Autodesk Fusion 360 part; units mm, degrees
(part 4 of 24)
  arc A1417 (34.9504, 19.1008) -> (35.0012, 19.1008) centre (34.9758, 19.1008) ccw
  arc A1418 (30.7467, 19.1982) -> (30.7975, 19.1982) centre (30.7721, 19.1982) ccw
  arc A1419 (40.8996, 22.1629) -> (40.8996, 22.2137) centre (40.8996, 22.1883) ccw
  arc A1420 (27.3478, 19.5144) -> (27.3638, 19.4662) centre (27.3558, 19.4903) ccw
  arc A1421 (32.4358, 19.1262) -> (32.4358, 19.0754) centre (32.4358, 19.1008) ccw
  arc A1422 (32.4104, 19.4254) -> (32.4612, 19.4254) centre (32.4358, 19.4254) ccw
  arc A1423 (32.8253, 20.2819) -> (33.0849, 20.5415) centre (32.8253, 20.5415) ccw
  line L436 (33.6042, 19.1008) -> (32.4358, 19.1008)
  arc A1424 (29.8878, 19.5144) -> (29.9038, 19.4662) centre (29.8958, 19.4903) ccw
  arc A1425 (32.8253, 20.3073) -> (32.8253, 20.2565) centre (32.8253, 20.2819) ccw
  arc A1426 (33.1103, 20.5415) -> (33.0595, 20.5415) centre (33.0849, 20.5415) ccw
  arc A1427 (32.8253, 20.2565) -> (32.8253, 20.3073) centre (32.8253, 20.2819) ccw
  line L437 (40.0558, 21.5392) -> (40.0558, 21.8637)
  arc A1428 (31.0642, 20.6333) -> (30.4151, 20.6333) centre (30.7396, 20.6333) ccw
  line L438 (31.0642, 20.3087) -> (31.0642, 20.6333)
  line L439 (33.6042, 19.4254) -> (33.6042, 19.1008)
  arc A1429 (27.3558, 20.6657) -> (27.6154, 20.3087) centre (27.731, 20.6657) ccw
  line L440 (41.2242, 21.8637) -> (41.2242, 21.5392)
  line L441 (29.8958, 19.4903) -> (31.0642, 19.8797)
  line L442 (30.4151, 20.6982) -> (30.4151, 20.4385)
  arc A1430 (31.0388, 20.6333) -> (31.0896, 20.6333) centre (31.0642, 20.6333) ccw
  arc A1431 (30.4405, 20.6982) -> (30.3897, 20.6982) centre (30.4151, 20.6982) ccw
  arc A1432 (33.6042, 19.4254) -> (33.2796, 19.7499) centre (33.2796, 19.4253) ccw
  arc A1433 (33.0595, 20.5415) -> (33.1103, 20.5415) centre (33.0849, 20.5415) ccw
  arc A1434 (32.7604, 19.7499) -> (32.4358, 19.4254) centre (32.7604, 19.4253) ccw
  arc A1435 (40.0304, 21.5392) -> (40.0812, 21.5392) centre (40.0558, 21.5392) ccw
  arc A1436 (30.4151, 20.6982) -> (29.8958, 20.6982) centre (30.1554, 20.6982) ccw
  arc A1437 (32.7604, 20.3073) -> (32.7604, 20.2565) centre (32.7604, 20.2819) ccw
  line L443 (32.7604, 19.7499) -> (33.2796, 19.7499)
  arc A1438 (33.5788, 19.1008) -> (33.6296, 19.1008) centre (33.6042, 19.1008) ccw
  line L444 (34.9758, 19.1008) -> (34.9758, 19.4254)
  arc A1439 (31.0722, 19.8556) -> (31.0562, 19.9038) centre (31.0642, 19.8797) ccw
  arc A1440 (30.3897, 20.6982) -> (30.4405, 20.6982) centre (30.4151, 20.6982) ccw
  arc A1441 (28.5496, 20.9578) -> (28.4988, 20.9578) centre (28.5242, 20.9578) ccw
  arc A1442 (33.2796, 19.7753) -> (33.2796, 19.7245) centre (33.2796, 19.7499) ccw
  arc A1443 (29.8704, 20.6982) -> (29.9212, 20.6982) centre (29.8958, 20.6982) ccw
  arc A1444 (32.4104, 19.1008) -> (32.4612, 19.1008) centre (32.4358, 19.1008) ccw
  arc A1445 (32.7604, 19.7245) -> (32.7604, 19.7753) centre (32.7604, 19.7499) ccw
  arc A1446 (33.0849, 20.9056) -> (33.0849, 20.9564) centre (33.0849, 20.931) ccw
  arc A1447 (29.8704, 20.3087) -> (29.9212, 20.3087) centre (29.8958, 20.3087) ccw
  arc A1448 (32.7604, 19.7753) -> (32.7604, 19.7245) centre (32.7604, 19.7499) ccw
  arc A1449 (30.7975, 19.7824) -> (30.7467, 19.7824) centre (30.7721, 19.7824) ccw
  line L445 (29.8958, 20.3087) -> (29.8958, 20.6982)
  line L446 (30.7721, 19.7824) -> (30.7721, 19.1982)
  arc A1450 (33.2796, 19.7245) -> (33.2796, 19.7753) centre (33.2796, 19.7499) ccw
  arc A1451 (31.0388, 20.3087) -> (31.0896, 20.3087) centre (31.0642, 20.3087) ccw
  arc A1452 (30.3897, 20.6333) -> (30.4405, 20.6333) centre (30.4151, 20.6333) ccw
  arc A1453 (32.7604, 20.931) -> (32.7604, 20.2819) centre (32.7604, 20.6065) ccw
  arc A1454 (35.0012, 19.4254) -> (34.9504, 19.4254) centre (34.9758, 19.4254) ccw
  line L447 (33.0849, 20.931) -> (33.0849, 20.5415)
  arc A1455 (29.9212, 20.6982) -> (29.8704, 20.6982) centre (29.8958, 20.6982) ccw
  line L448 (32.4358, 19.1008) -> (32.4358, 19.4254)
  arc A1456 (32.7604, 20.9056) -> (32.7604, 20.9564) centre (32.7604, 20.931) ccw
  arc A1457 (33.6296, 19.4254) -> (33.5788, 19.4254) centre (33.6042, 19.4254) ccw
  line L449 (36.1442, 20.2819) -> (36.1442, 20.931)
  arc A1458 (35.1269, 21.9995) -> (35.1492, 21.9538) centre (35.138, 21.9767) ccw
  arc A1459 (34.9956, 20.6223) -> (34.956, 20.5906) centre (34.9758, 20.6065) ccw
  arc A1460 (35.2513, 22.0289) -> (35.2196, 21.9893) centre (35.2355, 22.0091) ccw
  arc A1461 (35.1492, 21.5451) -> (35.1269, 21.4994) centre (35.138, 21.5223) ccw
  arc A1462 (35.9737, 21.5463) -> (35.9902, 21.4982) centre (35.9819, 21.5222) ccw
  arc A1463 (35.9902, 22.0007) -> (35.9737, 21.9526) centre (35.9819, 21.9767) ccw
  arc A1464 (38.2552, 25.0613) -> (38.2044, 25.0613) centre (38.2298, 25.0613) ccw
  line L450 (36.1442, 19.4254) -> (36.1442, 19.1008)
  arc A1465 (33.1103, 20.931) -> (33.0595, 20.931) centre (33.0849, 20.931) ccw
  arc A1466 (36.1188, 19.1008) -> (36.1696, 19.1008) centre (36.1442, 19.1008) ccw
  arc A1467 (35.8196, 19.7753) -> (35.8196, 19.7245) centre (35.8196, 19.7499) ccw
  arc A1468 (38.2552, 23.7659) -> (38.2044, 23.7659) centre (38.2298, 23.7659) ccw
  line L451 (38.2298, 24.2824) -> (38.2298, 25.0613)
  arc A1469 (33.5788, 19.4254) -> (33.6296, 19.4254) centre (33.6042, 19.4254) ccw
  arc A1470 (34.9758, 19.1262) -> (34.9758, 19.0754) centre (34.9758, 19.1008) ccw
  arc A1471 (36.1442, 19.0754) -> (36.1442, 19.1262) centre (36.1442, 19.1008) ccw
  line L452 (38.2298, 20.3962) -> (38.2298, 21.1751)
  line L453 (35.3004, 19.7499) -> (35.8196, 19.7499)
  arc A1472 (35.56, 21.4503) -> (35.56, 21.3995) centre (35.56, 21.4249) ccw
  arc A1473 (36.1188, 20.2819) -> (36.1696, 20.2819) centre (36.1442, 20.2819) ccw
  arc A1474 (35.8687, 21.47) -> (35.9004, 21.5096) centre (35.8845, 21.4898) ccw
  arc A1475 (38.2552, 19.8797) -> (38.2044, 19.8797) centre (38.2298, 19.8797) ccw
  arc A1476 (38.2044, 24.2824) -> (38.2552, 24.2824) centre (38.2298, 24.2824) ccw
  line L454 (38.2298, 22.987) -> (38.2298, 23.7659)
  arc A1477 (33.0849, 20.9564) -> (33.0849, 20.9056) centre (33.0849, 20.931) ccw
  arc A1478 (35.56, 22.074) -> (35.1381, 21.9766) centre (35.5601, 21.1113) ccw
  arc A1479 (35.0012, 21.7494) -> (34.9504, 21.7494) centre (34.9758, 21.7494) ccw
  arc A1480 (33.6042, 19.0754) -> (33.6042, 19.1262) centre (33.6042, 19.1008) ccw
  arc A1481 (34.9758, 20.6319) -> (34.9758, 20.5811) centre (34.9758, 20.6065) ccw
  arc A1482 (33.5788, 20.4117) -> (33.6296, 20.4117) centre (33.6042, 20.4117) ccw
  line L455 (34.9758, 20.6065) -> (36.1442, 20.6065)
  arc A1483 (34.9504, 21.7494) -> (35.0012, 21.7494) centre (34.9758, 21.7494) ccw
  arc A1484 (38.2044, 20.3962) -> (38.2552, 20.3962) centre (38.2298, 20.3962) ccw
  arc A1485 (36.1442, 21.7494) -> (35.9819, 21.9766) centre (35.904, 21.7494) ccw
  arc A1486 (35.1381, 21.9766) -> (34.9758, 21.7494) centre (35.216, 21.7494) ccw
  arc A1487 (36.1696, 21.7494) -> (36.1188, 21.7494) centre (36.1442, 21.7494) ccw
  arc A1488 (36.1442, 20.5811) -> (36.1442, 20.6319) centre (36.1442, 20.6065) ccw
  arc A1489 (35.1463, 21.9526) -> (35.1298, 22.0007) centre (35.138, 21.9766) ccw
  arc A1490 (35.9931, 21.4994) -> (35.9708, 21.5451) centre (35.982, 21.5223) ccw
  line L456 (32.8253, 20.2819) -> (32.7604, 20.2819)
  arc A1491 (35.56, 21.4249) -> (35.9819, 21.5223) centre (35.5599, 22.3876) ccw
  arc A1492 (36.1442, 19.4254) -> (35.8196, 19.7499) centre (35.8196, 19.4253) ccw
  arc A1493 (35.3004, 19.7753) -> (35.3004, 19.7245) centre (35.3004, 19.7499) ccw
  arc A1494 (35.56, 22.0994) -> (35.56, 22.0486) centre (35.56, 22.074) ccw
  line L457 (38.2298, 19.1008) -> (38.2298, 19.8797)
  arc A1495 (34.9504, 19.4254) -> (35.0012, 19.4254) centre (34.9758, 19.4254) ccw
  arc A1496 (36.1696, 20.931) -> (36.1188, 20.931) centre (36.1442, 20.931) ccw
  line L458 (76.7842, 35.6108) -> (75.6158, 36.0003)
  arc A1497 (35.9819, 21.5223) -> (36.1442, 21.7494) centre (35.9041, 21.7494) ccw
  arc A1498 (35.8196, 19.7245) -> (35.8196, 19.7753) centre (35.8196, 19.7499) ccw
  arc A1499 (36.1188, 21.7494) -> (36.1696, 21.7494) centre (36.1442, 21.7494) ccw
  arc A1500 (35.56, 22.0486) -> (35.56, 22.0994) centre (35.56, 22.074) ccw
  arc A1501 (75.6238, 36.0244) -> (75.6078, 35.9762) centre (75.6158, 36.0003) ccw
  arc A1502 (35.1381, 21.5223) -> (35.56, 21.4249) centre (35.5601, 22.3876) ccw
  arc A1503 (34.9758, 21.7494) -> (35.1381, 21.5223) centre (35.2159, 21.7494) ccw
  arc A1504 (35.1298, 21.4982) -> (35.1463, 21.5463) centre (35.1381, 21.5222) ccw
  line L459 (38.2298, 21.6916) -> (38.2298, 22.4705)
  arc A1505 (35.9819, 21.9766) -> (35.56, 22.074) centre (35.5599, 21.1113) ccw
  arc A1506 (36.1696, 19.4254) -> (36.1188, 19.4254) centre (36.1442, 19.4254) ccw
  arc A1507 (38.2044, 19.1008) -> (38.2552, 19.1008) centre (38.2298, 19.1008) ccw
  arc A1508 (35.9708, 21.9538) -> (35.9931, 21.9995) centre (35.9819, 21.9767) ccw
  arc A1509 (36.1188, 19.4254) -> (36.1696, 19.4254) centre (36.1442, 19.4254) ccw
  line L460 (36.1442, 19.1008) -> (34.9758, 19.1008)
  arc A1510 (75.9404, 40.6301) -> (75.6158, 40.3056) centre (75.9404, 40.3055) ccw
  arc A1511 (75.5904, 40.3056) -> (75.6412, 40.3056) centre (75.6158, 40.3056) ccw
  arc A1512 (75.6228, 37.1028) -> (75.6088, 37.0539) centre (75.6158, 37.0784) ccw
  arc A1513 (75.6412, 40.3056) -> (75.5904, 40.3056) centre (75.6158, 40.3056) ccw
  arc A1514 (75.7335, 39.407) -> (75.6928, 39.4374) centre (75.7132, 39.4222) ccw
  arc A1515 (76.4596, 40.6555) -> (76.4596, 40.6047) centre (76.4596, 40.6301) ccw
  arc A1516 (76.4992, 36.8187) -> (76.55, 36.8187) centre (76.5246, 36.8187) ccw
  arc A1517 (76.2649, 37.2985) -> (76.2649, 37.2477) centre (76.2649, 37.2731) ccw
  line L461 (75.6158, 36.0003) -> (76.7842, 36.3897)
  arc A1518 (75.9404, 40.6047) -> (75.9404, 40.6555) centre (75.9404, 40.6301) ccw
  line L462 (76.914, 37.9123) -> (75.486, 38.4316)
  arc A1519 (76.0803, 39.0124) -> (76.1249, 38.9881) centre (76.1026, 39.0003) ccw
  arc A1520 (38.2552, 21.1751) -> (38.2044, 21.1751) centre (38.2298, 21.1751) ccw
  line L463 (76.2649, 37.2731) -> (76.7842, 37.2731)
  arc A1521 (76.55, 37.4678) -> (76.4992, 37.4678) centre (76.5246, 37.4678) ccw
  arc A1522 (75.6078, 36.0244) -> (75.6238, 35.9762) centre (75.6158, 36.0003) ccw
  arc A1523 (75.8754, 38.8705) -> (76.1026, 39.0003) centre (75.8754, 39.1342) ccw
  arc A1524 (76.7588, 39.2275) -> (76.8096, 39.2275) centre (76.7842, 39.2275) ccw
  arc A1525 (76.8096, 39.2275) -> (76.7588, 39.2275) centre (76.7842, 39.2275) ccw
  arc A1526 (35.3004, 19.7245) -> (35.3004, 19.7753) centre (35.3004, 19.7499) ccw
  line L464 (76.2974, 39.3573) -> (76.1026, 39.0003)
  arc A1527 (38.2044, 21.6916) -> (38.2552, 21.6916) centre (38.2298, 21.6916) ccw
  arc A1528 (76.6219, 38.838) -> (76.7842, 39.2275) centre (76.2357, 39.2275) ccw
  arc A1529 (35.2156, 20.266) -> (35.2553, 20.2978) centre (35.2355, 20.2819) ccw
  arc A1530 (75.8754, 38.8959) -> (75.8754, 38.8451) centre (75.8754, 38.8705) ccw
  line L465 (76.7842, 39.981) -> (75.6158, 39.981)
  line L466 (75.6158, 41.4867) -> (76.7842, 41.8761)
  line L467 (75.6158, 37.0784) -> (76.5246, 36.8187)
  arc A1531 (76.7922, 41.852) -> (76.7762, 41.9002) centre (76.7842, 41.8761) ccw
  arc A1532 (75.4947, 38.4555) -> (75.4773, 38.4077) centre (75.486, 38.4316) ccw
  arc A1533 (75.6158, 39.1301) -> (75.8754, 38.8705) centre (75.8754, 39.1301) ccw
  arc A1534 (76.9053, 37.8884) -> (76.9227, 37.9362) centre (76.914, 37.9123) ccw
  arc A1535 (75.6412, 39.1301) -> (75.5904, 39.1301) centre (75.6158, 39.1301) ccw
  line L468 (35.8846, 21.4898) -> (35.2354, 22.0091)
  arc A1536 (38.2044, 22.987) -> (38.2552, 22.987) centre (38.2298, 22.987) ccw
  arc A1537 (76.4596, 40.6047) -> (76.4596, 40.6555) centre (76.4596, 40.6301) ccw
  arc A1538 (75.6158, 40.0064) -> (75.6158, 39.9556) centre (75.6158, 39.981) ccw
  arc A1539 (35.56, 21.3995) -> (35.56, 21.4503) centre (35.56, 21.4249) ccw
  arc A1540 (76.5246, 39.4871) -> (76.2974, 39.3573) centre (76.5246, 39.2234) ccw
  arc A1541 (76.7842, 39.2275) -> (76.5246, 39.4871) centre (76.5246, 39.2275) ccw
  arc A1542 (76.7922, 36.3656) -> (76.7762, 36.4138) centre (76.7842, 36.3897) ccw
  arc A1543 (75.9404, 40.6555) -> (75.9404, 40.6047) centre (75.9404, 40.6301) ccw
  line L469 (35.2354, 20.2819) -> (34.9758, 20.6065)
  arc A1544 (75.7132, 39.4222) -> (75.6158, 39.1301) centre (76.1026, 39.1301) ccw
  arc A1545 (76.7842, 39.9556) -> (76.7842, 40.0064) centre (76.7842, 39.981) ccw
  arc A1546 (76.7588, 40.3056) -> (76.8096, 40.3056) centre (76.7842, 40.3056) ccw
  arc A1547 (76.2755, 39.3702) -> (76.3193, 39.3444) centre (76.2974, 39.3573) ccw
  line L470 (76.7842, 40.3056) -> (76.7842, 39.981)
  arc A1548 (75.5904, 39.1301) -> (75.6412, 39.1301) centre (75.6158, 39.1301) ccw
  arc A1549 (76.604, 38.856) -> (76.6398, 38.82) centre (76.6219, 38.838) ccw
  line L471 (76.5246, 36.8187) -> (76.5246, 37.4678)
  arc A1550 (76.5246, 39.5125) -> (76.5246, 39.4617) centre (76.5246, 39.4871) ccw
  arc A1551 (76.7842, 37.2477) -> (76.7842, 37.2985) centre (76.7842, 37.2731) ccw
  arc A1552 (75.6078, 41.5108) -> (75.6238, 41.4626) centre (75.6158, 41.4867) ccw
  line L472 (75.6158, 39.981) -> (75.6158, 40.3056)
  line L473 (75.9404, 40.6301) -> (76.4596, 40.6301)
  arc A1553 (38.2552, 22.4705) -> (38.2044, 22.4705) centre (38.2298, 22.4705) ccw
  arc A1554 (75.5904, 39.981) -> (75.6412, 39.981) centre (75.6158, 39.981) ccw
  arc A1555 (76.4667, 35.7082) -> (76.5175, 35.7082) centre (76.4921, 35.7082) ccw
  arc A1556 (76.7762, 35.5867) -> (76.7922, 35.6349) centre (76.7842, 35.6108) ccw
  arc A1557 (76.5176, 36.7943) -> (76.5315, 36.8431) centre (76.5246, 36.8187) ccw
  arc A1558 (76.5175, 36.2924) -> (76.4667, 36.2924) centre (76.4921, 36.2924) ccw
  line L474 (76.4921, 36.2924) -> (76.4921, 35.7082)
  arc A1559 (75.8754, 38.8451) -> (75.8754, 38.8959) centre (75.8754, 38.8705) ccw
  arc A1560 (76.7762, 41.0731) -> (76.7922, 41.1213) centre (76.7842, 41.0972) ccw
  arc A1561 (76.4667, 41.1946) -> (76.5175, 41.1946) centre (76.4921, 41.1946) ccw
  arc A1562 (79.3496, 40.1992) -> (79.2988, 40.1992) centre (79.3242, 40.1992) ccw
  arc A1563 (79.3242, 39.2275) -> (79.0646, 39.4871) centre (79.0646, 39.2275) ccw
  arc A1564 (78.6497, 36.8187) -> (78.7005, 36.8187) centre (78.6751, 36.8187) ccw
  arc A1565 (76.7842, 40.3056) -> (76.4596, 40.6301) centre (76.4596, 40.3055) ccw
  arc A1566 (76.8096, 40.3056) -> (76.7588, 40.3056) centre (76.7842, 40.3056) ccw
  arc A1567 (78.9347, 37.4932) -> (78.9347, 37.4424) centre (78.9347, 37.4678) ccw
  arc A1568 (79.4453, 37.8884) -> (79.4627, 37.9362) centre (79.454, 37.9123) ccw
  arc A1569 (79.0646, 39.965) -> (79.0646, 39.9142) centre (79.0646, 39.9396) ccw
  line L475 (78.1558, 36.8187) -> (78.1558, 37.4678)
  line L476 (79.0321, 36.2924) -> (79.0321, 35.7082)
  arc A1570 (79.3322, 36.3656) -> (79.3162, 36.4138) centre (79.3242, 36.3897) ccw
  arc A1571 (78.9347, 37.4678) -> (78.6751, 37.2082) centre (78.9347, 37.2082) ccw
  arc A1572 (78.6751, 36.7933) -> (78.6751, 36.8441) centre (78.6751, 36.8187) ccw
  arc A1573 (79.0646, 37.4932) -> (79.0646, 37.4424) centre (79.0646, 37.4678) ccw
  arc A1574 (79.2988, 37.2082) -> (79.3496, 37.2082) centre (79.3242, 37.2082) ccw
  line L477 (78.8374, 39.3573) -> (78.6426, 39.0003)
  line L478 (79.3242, 40.4589) -> (79.3242, 40.1992)
  arc A1575 (76.5175, 41.7788) -> (76.4667, 41.7788) centre (76.4921, 41.7788) ccw
  arc A1576 (76.1245, 38.9874) -> (76.0808, 39.0132) centre (76.1026, 39.0003) ccw
  arc A1577 (75.6238, 41.5108) -> (75.6078, 41.4626) centre (75.6158, 41.4867) ccw
  arc A1578 (78.8597, 39.3451) -> (78.8151, 39.3695) centre (78.8374, 39.3573) ccw
  arc A1579 (79.3242, 37.2082) -> (79.0646, 37.4678) centre (79.0646, 37.2082) ccw
  arc A1580 (78.1478, 36.0244) -> (78.1638, 35.9762) centre (78.1558, 36.0003) ccw
  line L479 (78.6751, 36.8187) -> (78.1558, 36.8187)
  line L480 (78.1558, 36.0003) -> (79.3242, 36.3897)
  arc A1581 (78.0347, 38.4555) -> (78.0173, 38.4077) centre (78.026, 38.4316) ccw
  arc A1582 (79.0646, 39.9396) -> (79.3242, 40.1992) centre (79.0646, 40.1992) ccw
  line L481 (79.0646, 37.4678) -> (78.9347, 37.4678)
  arc A1583 (76.5246, 39.4617) -> (76.5246, 39.5125) centre (76.5246, 39.4871) ccw
  arc A1584 (79.1619, 38.838) -> (79.3242, 39.2275) centre (78.7757, 39.2275) ccw
  line L482 (79.0646, 39.9396) -> (78.4154, 39.9396)
  arc A1585 (78.1304, 39.1301) -> (78.1812, 39.1301) centre (78.1558, 39.1301) ccw
  arc A1586 (79.0646, 37.4424) -> (79.0646, 37.4932) centre (79.0646, 37.4678) ccw
  line L483 (76.4921, 41.7788) -> (76.4921, 41.1946)
  arc A1587 (79.144, 38.856) -> (79.1798, 38.82) centre (79.1619, 38.838) ccw
  arc A1588 (79.3162, 35.5867) -> (79.3322, 35.6349) centre (79.3242, 35.6108) ccw
  arc A1589 (78.4154, 38.8451) -> (78.4154, 38.8959) centre (78.4154, 38.8705) ccw
  arc A1590 (76.7588, 39.981) -> (76.8096, 39.981) centre (76.7842, 39.981) ccw
  arc A1591 (79.0575, 36.2924) -> (79.0067, 36.2924) centre (79.0321, 36.2924) ccw
  arc A1592 (78.1304, 36.8187) -> (78.1812, 36.8187) centre (78.1558, 36.8187) ccw
  arc A1593 (78.1812, 39.1301) -> (78.1304, 39.1301) centre (78.1558, 39.1301) ccw
  arc A1594 (79.0646, 39.4617) -> (79.0646, 39.5125) centre (79.0646, 39.4871) ccw
  arc A1595 (79.2988, 40.1992) -> (79.3496, 40.1992) centre (79.3242, 40.1992) ccw
  line L484 (78.6751, 37.2082) -> (78.6751, 36.8187)
  arc A1596 (78.2532, 39.4222) -> (78.1558, 39.1301) centre (78.6426, 39.1301) ccw
  arc A1597 (76.3197, 39.3451) -> (76.2751, 39.3695) centre (76.2974, 39.3573) ccw
  arc A1598 (78.1812, 37.4678) -> (78.1304, 37.4678) centre (78.1558, 37.4678) ccw
  arc A1599 (78.1638, 36.0244) -> (78.1478, 35.9762) centre (78.1558, 36.0003) ccw
  arc A1600 (79.0646, 39.4871) -> (78.8374, 39.3573) centre (79.0646, 39.2234) ccw
  arc A1601 (79.3496, 37.2082) -> (79.2988, 37.2082) centre (79.3242, 37.2082) ccw
  arc A1602 (78.6497, 37.2082) -> (78.7005, 37.2082) centre (78.6751, 37.2082) ccw
  arc A1603 (78.1558, 39.1301) -> (78.4154, 38.8705) centre (78.4154, 39.1301) ccw
  arc A1604 (79.0067, 35.7082) -> (79.0575, 35.7082) centre (79.0321, 35.7082) ccw
  arc A1605 (79.3496, 39.2275) -> (79.2988, 39.2275) centre (79.3242, 39.2275) ccw
  arc A1606 (79.2988, 36.8187) -> (79.3496, 36.8187) centre (79.3242, 36.8187) ccw
  line L485 (79.454, 37.9123) -> (78.026, 38.4316)
  arc A1607 (79.2988, 39.2275) -> (79.3496, 39.2275) centre (79.3242, 39.2275) ccw
  arc A1608 (78.6645, 38.9874) -> (78.6208, 39.0132) centre (78.6427, 39.0003) ccw
  arc A1609 (78.2735, 39.407) -> (78.2328, 39.4374) centre (78.2532, 39.4222) ccw
  line L486 (76.7842, 41.0972) -> (75.6158, 41.4867)
  arc A1610 (78.4154, 38.8705) -> (78.6426, 39.0003) centre (78.4154, 39.1342) ccw
  arc A1611 (78.9347, 37.4424) -> (78.9347, 37.4932) centre (78.9347, 37.4678) ccw
  line L487 (79.3242, 36.8187) -> (79.3242, 37.2082)
  arc A1612 (81.8642, 39.6437) -> (81.5396, 39.9683) centre (81.5396, 39.6437) ccw
  arc A1613 (81.8642, 38.0746) -> (81.8642, 38.1254) centre (81.8642, 38.1) ccw
  arc A1614 (80.6704, 37.1404) -> (80.7212, 37.1404) centre (80.6958, 37.1404) ccw
  arc A1615 (78.7005, 37.2082) -> (78.6497, 37.2082) centre (78.6751, 37.2082) ccw
  arc A1616 (81.8896, 37.1404) -> (81.8388, 37.1404) centre (81.8642, 37.1404) ccw
  line L488 (81.6046, 36.8808) -> (80.9554, 36.8808)
  arc A1617 (81.8896, 37.5299) -> (81.8388, 37.5299) centre (81.8642, 37.5299) ccw
  arc A1618 (81.8642, 39.2938) -> (81.8642, 39.3446) centre (81.8642, 39.3192) ccw
  line L489 (79.3242, 35.6108) -> (78.1558, 36.0003)
  arc A1619 (78.1558, 36.8441) -> (78.1558, 36.7933) centre (78.1558, 36.8187) ccw
  arc A1620 (78.8155, 39.3702) -> (78.8593, 39.3444) centre (78.8374, 39.3573) ccw
  arc A1621 (81.8896, 39.6437) -> (81.8388, 39.6437) centre (81.8642, 39.6437) ccw
  arc A1622 (78.1558, 40.1992) -> (78.4154, 39.9396) centre (78.4154, 40.1992) ccw
  arc A1623 (81.1897, 37.3352) -> (81.2405, 37.3352) centre (81.2151, 37.3352) ccw
  arc A1624 (81.8765, 38.7269) -> (81.8519, 38.7713) centre (81.8642, 38.7491) ccw
  arc A1625 (81.5396, 39.9937) -> (81.5396, 39.9429) centre (81.5396, 39.9683) ccw
  arc A1626 (81.8642, 37.5045) -> (81.8642, 37.5553) centre (81.8642, 37.5299) ccw
  arc A1627 (79.2988, 40.9358) -> (79.3496, 40.9358) centre (79.3242, 40.9358) ccw
  line L490 (78.1558, 40.9358) -> (79.3242, 40.9358)
  arc A1628 (80.6958, 38.7745) -> (80.6958, 38.7237) centre (80.6958, 38.7491) ccw
  arc A1629 (78.1304, 40.1992) -> (78.1812, 40.1992) centre (78.1558, 40.1992) ccw
  arc A1630 (80.7212, 37.1404) -> (80.6704, 37.1404) centre (80.6958, 37.1404) ccw
  line L491 (80.6958, 39.3192) -> (80.6958, 39.6437)
  arc A1631 (79.3496, 41.455) -> (79.2988, 41.455) centre (79.3242, 41.455) ccw
  arc A1632 (78.1812, 40.4589) -> (78.1304, 40.4589) centre (78.1558, 40.4589) ccw
  arc A1633 (81.8642, 38.7237) -> (81.8642, 38.7745) centre (81.8642, 38.7491) ccw
  arc A1634 (80.6835, 38.1222) -> (80.7081, 38.0778) centre (80.6958, 38.1) ccw
  arc A1635 (81.2405, 37.5299) -> (81.1897, 37.5299) centre (81.2151, 37.5299) ccw
  arc A1636 (81.6046, 36.8808) -> (81.8642, 37.1404) centre (81.6046, 37.1404) ccw
  arc A1637 (78.4154, 39.9142) -> (78.4154, 39.965) centre (78.4154, 39.9396) ccw
  arc A1638 (80.6704, 39.6437) -> (80.7212, 39.6437) centre (80.6958, 39.6437) ccw
  line L492 (81.8642, 39.6437) -> (81.8642, 39.3192)
  arc A1639 (81.2151, 37.5553) -> (81.2151, 37.5045) centre (81.2151, 37.5299) ccw
  line L493 (81.8642, 39.3192) -> (80.6958, 39.3192)
  line L494 (81.8642, 38.7491) -> (80.6958, 38.7491)
  arc A1640 (80.9554, 36.8554) -> (80.9554, 36.9062) centre (80.9554, 36.8808) ccw
  line L495 (80.6958, 38.1) -> (81.8642, 38.7491)
  arc A1641 (78.1558, 40.9612) -> (78.1558, 40.9104) centre (78.1558, 40.9358) ccw
  arc A1642 (79.3242, 40.9104) -> (79.3242, 40.9612) centre (79.3242, 40.9358) ccw
  arc A1643 (81.6046, 36.8554) -> (81.6046, 36.9062) centre (81.6046, 36.8808) ccw
  line L496 (81.8642, 38.1) -> (80.6958, 38.1)
  line L497 (78.1558, 40.1992) -> (78.1558, 40.4589)
  arc A1644 (80.7212, 39.6437) -> (80.6704, 39.6437) centre (80.6958, 39.6437) ccw
  arc A1645 (81.0204, 39.9683) -> (80.6958, 39.6437) centre (81.0204, 39.6437) ccw
  arc A1646 (81.8388, 37.1404) -> (81.8896, 37.1404) centre (81.8642, 37.1404) ccw
  line L498 (81.2151, 37.3352) -> (81.2151, 37.5299)
  arc A1647 (81.8388, 39.3192) -> (81.8896, 39.3192) centre (81.8642, 39.3192) ccw
  arc A1648 (79.0646, 39.9142) -> (79.0646, 39.965) centre (79.0646, 39.9396) ccw
  arc A1649 (81.6046, 36.9062) -> (81.6046, 36.8554) centre (81.6046, 36.8808) ccw
  arc A1650 (78.4154, 38.8959) -> (78.4154, 38.8451) centre (78.4154, 38.8705) ccw
  arc A1651 (79.0646, 39.5125) -> (79.0646, 39.4617) centre (79.0646, 39.4871) ccw
  arc A1652 (78.6203, 39.0124) -> (78.6649, 38.9881) centre (78.6426, 39.0003) ccw
  arc A1653 (80.6958, 37.1404) -> (80.9554, 36.8808) centre (80.9554, 37.1404) ccw
  arc A1654 (73.8152, 37.6597) -> (73.7644, 37.6597) centre (73.7898, 37.6597) ccw
  arc A1655 (78.4154, 39.965) -> (78.4154, 39.9142) centre (78.4154, 39.9396) ccw
  line L499 (79.3242, 40.9358) -> (79.3242, 41.455)
  arc A1656 (79.3496, 40.4589) -> (79.2988, 40.4589) centre (79.3242, 40.4589) ccw
  arc A1657 (80.7212, 37.5299) -> (80.6704, 37.5299) centre (80.6958, 37.5299) ccw
  line L500 (73.7898, 36.8808) -> (73.7898, 37.6597)
  arc A1658 (81.8388, 39.6437) -> (81.8896, 39.6437) centre (81.8642, 39.6437) ccw
  arc A1659 (80.6958, 39.3446) -> (80.6958, 39.2938) centre (80.6958, 39.3192) ccw
  line L501 (81.8642, 37.5299) -> (81.8642, 37.1404)
  arc A1660 (81.5396, 39.9429) -> (81.5396, 39.9937) centre (81.5396, 39.9683) ccw
  arc A1661 (4.0462, 47.7012) -> (3.9954, 47.7012) centre (4.0208, 47.7012) ccw
  arc A1662 (5.5307, 46.5074) -> (5.5307, 46.5582) centre (5.5307, 46.5328) ccw
  arc A1663 (80.6958, 38.1254) -> (80.6958, 38.0746) centre (80.6958, 38.1) ccw
  line L502 (80.6958, 37.1404) -> (80.6958, 37.5299)
  line L503 (73.0758, 38.1649) -> (73.0758, 38.814)
  line L504 (73.0758, 39.243) -> (74.2442, 39.6325)
  arc A1664 (73.5697, 38.1649) -> (73.6205, 38.1649) centre (73.5951, 38.1649) ccw
  arc A1665 (74.2188, 38.5544) -> (74.2696, 38.5544) centre (74.2442, 38.5544) ccw
  arc A1666 (2.8448, 47.7266) -> (2.8448, 47.6758) centre (2.8448, 47.7012) ccw
  line L505 (3.1694, 47.0521) -> (2.8448, 47.0521)
  arc A1667 (73.0758, 38.1903) -> (73.0758, 38.1395) centre (73.0758, 38.1649) ccw
  arc A1668 (73.8547, 38.8394) -> (73.8547, 38.7886) centre (73.8547, 38.814) ccw
  arc A1669 (73.9846, 38.7886) -> (73.9846, 38.8394) centre (73.9846, 38.814) ccw
  arc A1670 (3.1694, 47.0521) -> (3.1694, 47.7012) centre (3.1694, 47.3767) ccw
  arc A1671 (3.1694, 47.7266) -> (3.1694, 47.6758) centre (3.1694, 47.7012) ccw
  arc A1672 (2.8448, 47.0775) -> (2.8448, 47.0267) centre (2.8448, 47.0521) ccw
  line L506 (74.2442, 39.6325) -> (73.0758, 40.0219)
  arc A1673 (73.4004, 37.2957) -> (73.4004, 37.2449) centre (73.4004, 37.2703) ccw
  arc A1674 (81.0204, 39.9429) -> (81.0204, 39.9937) centre (81.0204, 39.9683) ccw
  arc A1675 (4.5401, 47.6758) -> (4.5401, 47.7266) centre (4.5401, 47.7012) ccw
  arc A1676 (4.4103, 47.1565) -> (4.4103, 47.2073) centre (4.4103, 47.1819) ccw
  arc A1677 (2.8702, 47.7012) -> (2.8194, 47.7012) centre (2.8448, 47.7012) ccw
  arc A1678 (3.1694, 47.0775) -> (3.1694, 47.0267) centre (3.1694, 47.0521) ccw
  line L507 (5.0114, 46.5328) -> (5.5307, 46.5328)
  arc A1679 (78.1812, 40.1992) -> (78.1304, 40.1992) centre (78.1558, 40.1992) ccw
  arc A1680 (4.0208, 47.7266) -> (4.0208, 47.6758) centre (4.0208, 47.7012) ccw
  line L508 (4.5401, 46.5328) -> (4.0208, 46.5328)
  line L509 (74.1793, 37.2703) -> (73.4004, 37.2703)
  arc A1681 (73.9846, 38.8394) -> (73.9846, 38.7886) centre (73.9846, 38.814) ccw
  arc A1682 (74.2362, 39.6084) -> (74.2522, 39.6566) centre (74.2442, 39.6325) ccw
  arc A1683 (73.8547, 38.7886) -> (73.8547, 38.8394) centre (73.8547, 38.814) ccw
  arc A1684 (80.6704, 39.3192) -> (80.7212, 39.3192) centre (80.6958, 39.3192) ccw
  arc A1685 (81.0204, 39.9937) -> (81.0204, 39.9429) centre (81.0204, 39.9683) ccw
  arc A1686 (73.1012, 38.814) -> (73.0504, 38.814) centre (73.0758, 38.814) ccw
  arc A1687 (3.9954, 46.5328) -> (4.0462, 46.5328) centre (4.0208, 46.5328) ccw
  line L510 (4.0208, 46.5328) -> (4.0208, 47.7012)
  arc A1688 (3.257, 47.0634) -> (3.2115, 47.0407) centre (3.2343, 47.0521) ccw
  arc A1689 (74.2442, 38.5544) -> (73.9846, 38.814) centre (73.9846, 38.5544) ccw
  arc A1690 (3.4712, 46.5214) -> (3.5166, 46.5442) centre (3.4939, 46.5328) ccw
  arc A1691 (73.0838, 40.046) -> (73.0678, 39.9978) centre (73.0758, 40.0219) ccw
  arc A1692 (3.1694, 47.0267) -> (3.1694, 47.0775) centre (3.1694, 47.0521) ccw
  arc A1693 (2.8194, 46.5328) -> (2.8702, 46.5328) centre (2.8448, 46.5328) ccw
  line L511 (74.2442, 38.1649) -> (74.2442, 38.5544)
  line L512 (4.0208, 47.7012) -> (4.5401, 47.7012)
  arc A1694 (74.1793, 37.2449) -> (74.1793, 37.2957) centre (74.1793, 37.2703) ccw
  arc A1695 (74.2188, 38.1649) -> (74.2696, 38.1649) centre (74.2442, 38.1649) ccw
  arc A1696 (73.8547, 38.814) -> (73.5951, 38.5544) centre (73.8547, 38.5544) ccw
  arc A1697 (4.5401, 46.5074) -> (4.5401, 46.5582) centre (4.5401, 46.5328) ccw
  line L513 (81.0204, 39.9683) -> (81.5396, 39.9683)
  line L514 (2.8448, 47.7012) -> (3.1694, 47.7012)
  arc A1698 (80.9554, 36.9062) -> (80.9554, 36.8554) centre (80.9554, 36.8808) ccw
  line L515 (81.2151, 37.5299) -> (81.8642, 37.5299)
  arc A1699 (4.0208, 47.2073) -> (4.0208, 47.1565) centre (4.0208, 47.1819) ccw
  arc A1700 (5.0368, 47.7012) -> (4.986, 47.7012) centre (5.0114, 47.7012) ccw
  arc A1701 (74.2696, 38.5544) -> (74.2188, 38.5544) centre (74.2442, 38.5544) ccw
  arc A1702 (73.5697, 38.5544) -> (73.6205, 38.5544) centre (73.5951, 38.5544) ccw
  arc A1703 (73.6205, 38.5544) -> (73.5697, 38.5544) centre (73.5951, 38.5544) ccw
  arc A1704 (74.2522, 39.6084) -> (74.2362, 39.6566) centre (74.2442, 39.6325) ccw
  arc A1705 (5.0114, 46.5582) -> (5.0114, 46.5074) centre (5.0114, 46.5328) ccw
  line L516 (4.0208, 47.1819) -> (4.4103, 47.1819)
  arc A1706 (73.5951, 38.1395) -> (73.5951, 38.1903) centre (73.5951, 38.1649) ccw
  arc A1707 (73.0504, 38.1649) -> (73.1012, 38.1649) centre (73.0758, 38.1649) ccw
  line L517 (3.4939, 46.5328) -> (3.2343, 47.0521)
  arc A1708 (4.0208, 46.5582) -> (4.0208, 46.5074) centre (4.0208, 46.5328) ccw
  arc A1709 (21.0058, 53.8311) -> (21.0058, 53.7803) centre (21.0058, 53.8057) ccw
  arc A1710 (22.1865, 55.0605) -> (22.1619, 55.1049) centre (22.1742, 55.0827) ccw
  arc A1711 (18.8327, 52.4482) -> (18.8835, 52.4482) centre (18.8581, 52.4482) ccw
  arc A1712 (18.8835, 52.6429) -> (18.8327, 52.6429) centre (18.8581, 52.6429) ccw
  arc A1713 (5.9941, 46.8503) -> (5.9941, 46.7995) centre (5.9941, 46.8249) ccw
  arc A1714 (7.4084, 47.1641) -> (7.4499, 47.1348) centre (7.4292, 47.1495) ccw
  line L518 (5.0114, 47.7012) -> (5.0114, 46.5328)
  line L519 (73.9846, 38.814) -> (73.8547, 38.814)
  line L520 (22.1742, 52.8913) -> (21.0058, 53.2807)
  arc A1715 (20.9804, 53.6758) -> (21.0312, 53.6758) centre (21.0058, 53.6758) ccw
  arc A1716 (21.0058, 55.1081) -> (21.0058, 55.0573) centre (21.0058, 55.0827) ccw
  arc A1717 (5.8726, 46.5408) -> (5.9208, 46.5248) centre (5.8967, 46.5328) ccw
  line L521 (18.8581, 52.4482) -> (18.8581, 52.6429)
  arc A1718 (22.1742, 54.4082) -> (22.1742, 54.459) centre (22.1742, 54.4336) ccw
  line L522 (19.2476, 51.9938) -> (18.5984, 51.9938)
  arc A1719 (7.4084, 47.1348) -> (7.4499, 47.1641) centre (7.4291, 47.1494) ccw
  line L523 (21.0058, 52.5018) -> (22.1742, 52.8913)
  arc A1720 (7.8394, 47.6866) -> (7.7979, 47.7158) centre (7.8187, 47.7012) ccw
  line L524 (7.4292, 46.5328) -> (7.4292, 47.1495)
  arc A1721 (7.4546, 47.1495) -> (7.4038, 47.1495) centre (7.4292, 47.1495) ccw
  arc A1722 (22.1742, 55.0573) -> (22.1742, 55.1081) centre (22.1742, 55.0827) ccw
  arc A1723 (18.3642, 52.2534) -> (18.3134, 52.2534) centre (18.3388, 52.2534) ccw
  arc A1724 (19.4818, 52.2534) -> (19.5326, 52.2534) centre (19.5072, 52.2534) ccw
  arc A1725 (19.5326, 52.2534) -> (19.4818, 52.2534) centre (19.5072, 52.2534) ccw
  arc A1726 (18.3642, 52.6429) -> (18.3134, 52.6429) centre (18.3388, 52.6429) ccw
  arc A1727 (22.1996, 53.9355) -> (22.1488, 53.9355) centre (22.1742, 53.9355) ccw
  line L525 (7.4292, 47.1495) -> (7.8187, 47.7012)
  arc A1728 (4.986, 46.5328) -> (5.0368, 46.5328) centre (5.0114, 46.5328) ccw
  arc A1729 (20.9935, 54.4558) -> (21.0181, 54.4114) centre (21.0058, 54.4336) ccw
  arc A1730 (21.0138, 53.3048) -> (20.9978, 53.2566) centre (21.0058, 53.2807) ccw
  arc A1731 (19.2476, 51.9684) -> (19.2476, 52.0192) centre (19.2476, 51.9938) ccw
  arc A1732 (6.3103, 47.7092) -> (6.2621, 47.6932) centre (6.2862, 47.7012) ccw
  arc A1733 (19.2476, 51.9938) -> (19.5072, 52.2534) centre (19.2476, 52.2534) ccw
  line L526 (73.5951, 38.5544) -> (73.5951, 38.1649)
  line L527 (73.5951, 38.1649) -> (73.0758, 38.1649)
  arc A1734 (18.3134, 52.2534) -> (18.3642, 52.2534) centre (18.3388, 52.2534) ccw
  line L528 (6.5783, 46.8249) -> (5.9941, 46.8249)
  line L529 (7.0397, 47.7012) -> (7.4292, 47.1495)
  line L530 (18.3388, 52.2534) -> (18.3388, 52.6429)
  arc A1735 (21.0312, 53.9355) -> (20.9804, 53.9355) centre (21.0058, 53.9355) ccw
  arc A1736 (18.8581, 52.6683) -> (18.8581, 52.6175) centre (18.8581, 52.6429) ccw
  line L531 (18.8581, 52.6429) -> (19.5072, 52.6429)
  arc A1737 (22.1488, 53.6758) -> (22.1996, 53.6758) centre (22.1742, 53.6758) ccw
  line L532 (22.1742, 55.0827) -> (21.0058, 55.0827)
  line L533 (21.0058, 53.8057) -> (22.1742, 53.8057)
  line L534 (5.8967, 46.5328) -> (6.2862, 47.7012)
  line L535 (21.0058, 53.6758) -> (21.0058, 53.9355)
  arc A1738 (3.1694, 47.6758) -> (3.1694, 47.7266) centre (3.1694, 47.7012) ccw
  line L536 (19.5072, 52.6429) -> (19.5072, 52.2534)
  arc A1739 (20.9978, 52.5259) -> (21.0138, 52.4777) centre (21.0058, 52.5018) ccw
  arc A1740 (73.7644, 36.8808) -> (73.8152, 36.8808) centre (73.7898, 36.8808) ccw
  arc A1741 (19.2476, 52.0192) -> (19.2476, 51.9684) centre (19.2476, 51.9938) ccw
  arc A1742 (6.5783, 46.7995) -> (6.5783, 46.8503) centre (6.5783, 46.8249) ccw
  line L537 (2.8448, 46.5328) -> (2.8448, 47.7012)
  arc A1743 (18.5984, 52.0192) -> (18.5984, 51.9684) centre (18.5984, 51.9938) ccw
  line L538 (6.2862, 47.7012) -> (6.6757, 46.5328)
  arc A1744 (21.0058, 54.459) -> (21.0058, 54.4082) centre (21.0058, 54.4336) ccw
  arc A1745 (19.5326, 52.6429) -> (19.4818, 52.6429) centre (19.5072, 52.6429) ccw
  line L539 (22.1742, 54.4336) -> (21.0058, 54.4336)
  arc A1746 (18.5984, 51.9684) -> (18.5984, 52.0192) centre (18.5984, 51.9938) ccw
  arc A1747 (73.0678, 39.2671) -> (73.0838, 39.2189) centre (73.0758, 39.243) ccw
  arc A1748 (19.5072, 52.6175) -> (19.5072, 52.6683) centre (19.5072, 52.6429) ccw
  line L540 (19.5072, 53.213) -> (18.3388, 53.213)
  arc A1749 (22.1742, 53.7803) -> (22.1742, 53.8311) centre (22.1742, 53.8057) ccw
  arc A1750 (14.1676, 51.9684) -> (14.1676, 52.0192) centre (14.1676, 51.9938) ccw
  line L541 (22.1742, 53.6758) -> (22.1742, 53.9355)
  arc A1751 (18.3388, 53.8875) -> (18.3388, 53.8367) centre (18.3388, 53.8621) ccw
  arc A1752 (14.4272, 54.983) -> (14.4272, 55.0338) centre (14.4272, 55.0084) ccw
  arc A1753 (13.2334, 52.2534) -> (13.2842, 52.2534) centre (13.2588, 52.2534) ccw
  arc A1754 (19.5326, 54.7567) -> (19.4818, 54.7567) centre (19.5072, 54.7567) ccw
  arc A1755 (7.0605, 47.7158) -> (7.019, 47.6866) centre (7.0398, 47.7012) ccw
  arc A1756 (18.3388, 53.2384) -> (18.3388, 53.1876) centre (18.3388, 53.213) ccw
  arc A1757 (18.3265, 53.2352) -> (18.3511, 53.1908) centre (18.3388, 53.213) ccw
  arc A1758 (19.4818, 54.7567) -> (19.5326, 54.7567) centre (19.5072, 54.7567) ccw
  arc A1759 (18.3134, 54.7567) -> (18.3642, 54.7567) centre (18.3388, 54.7567) ccw
  arc A1760 (13.2588, 55.0338) -> (13.2588, 54.983) centre (13.2588, 55.0084) ccw
  line L542 (18.6634, 55.0813) -> (19.1826, 55.0813)
  arc A1761 (14.4526, 52.5131) -> (14.4018, 52.5131) centre (14.4272, 52.5131) ccw
  arc A1762 (13.2457, 53.0208) -> (13.2719, 52.9772) centre (13.2588, 52.999) ccw
  arc A1763 (19.5072, 53.1876) -> (19.5072, 53.2384) centre (19.5072, 53.213) ccw
  arc A1764 (7.4038, 46.5328) -> (7.4546, 46.5328) centre (7.4292, 46.5328) ccw
  arc A1765 (18.3642, 54.7567) -> (18.3134, 54.7567) centre (18.3388, 54.7567) ccw
  arc A1766 (18.3134, 54.4322) -> (18.3642, 54.4322) centre (18.3388, 54.4322) ccw
  arc A1767 (18.6634, 55.1067) -> (18.6634, 55.0559) centre (18.6634, 55.0813) ccw
  arc A1768 (18.6634, 55.0813) -> (18.3388, 54.7567) centre (18.6634, 54.7567) ccw
  line L543 (21.0058, 54.4336) -> (22.1742, 55.0827)
  arc A1769 (11.8618, 52.2534) -> (11.9126, 52.2534) centre (11.8872, 52.2534) ccw
  arc A1770 (19.5072, 53.8367) -> (19.5072, 53.8875) centre (19.5072, 53.8621) ccw
  line L544 (14.1676, 51.9938) -> (13.5184, 51.9938)
  arc A1771 (6.3103, 47.6932) -> (6.2621, 47.7092) centre (6.2862, 47.7012) ccw
  arc A1772 (13.2842, 52.5131) -> (13.2334, 52.5131) centre (13.2588, 52.5131) ccw
  arc A1773 (13.2588, 53.8033) -> (13.2588, 53.7525) centre (13.2588, 53.7779) ccw
  line L545 (18.3388, 53.213) -> (19.5072, 53.8621)
  arc A1774 (13.5184, 52.0192) -> (13.5184, 51.9684) centre (13.5184, 51.9938) ccw
  line L546 (11.8872, 52.5131) -> (11.8872, 52.2534)
  arc A1775 (19.5072, 54.4068) -> (19.5072, 54.4576) centre (19.5072, 54.4322) ccw
  arc A1776 (14.4018, 52.2534) -> (14.4526, 52.2534) centre (14.4272, 52.2534) ccw
  arc A1777 (14.1676, 51.9938) -> (14.4272, 52.2534) centre (14.1676, 52.2534) ccw
  line L547 (13.2588, 52.999) -> (13.9079, 53.3885)
  arc A1778 (14.4272, 54.3339) -> (14.4272, 54.3847) centre (14.4272, 54.3593) ccw
  line L548 (19.5072, 53.8621) -> (18.3388, 53.8621)
  arc A1779 (22.1822, 52.8672) -> (22.1662, 52.9154) centre (22.1742, 52.8913) ccw
  line L549 (19.5072, 54.7567) -> (19.5072, 54.4322)
  arc A1780 (22.1662, 52.8672) -> (22.1822, 52.9154) centre (22.1742, 52.8913) ccw
  arc A1781 (18.3388, 52.2534) -> (18.5984, 51.9938) centre (18.5984, 52.2534) ccw
  line L550 (14.4272, 52.999) -> (13.2588, 52.999)
  arc A1782 (13.921, 53.3667) -> (13.8948, 53.4103) centre (13.9079, 53.3885) ccw
  arc A1783 (19.5195, 53.8399) -> (19.4949, 53.8843) centre (19.5072, 53.8621) ccw
  arc A1784 (19.5072, 54.7567) -> (19.1826, 55.0813) centre (19.1826, 54.7567) ccw
  arc A1785 (19.1826, 55.1067) -> (19.1826, 55.0559) centre (19.1826, 55.0813) ccw
  arc A1786 (13.2588, 53.0244) -> (13.2588, 52.9736) centre (13.2588, 52.999) ccw
  line L551 (13.2588, 53.7779) -> (14.4272, 53.7779)
  arc A1787 (14.4272, 53.7525) -> (14.4272, 53.8033) centre (14.4272, 53.7779) ccw
  arc A1788 (18.6634, 55.0559) -> (18.6634, 55.1067) centre (18.6634, 55.0813) ccw
  line L552 (18.3388, 54.4322) -> (18.3388, 54.7567)
  arc A1789 (18.3388, 54.4576) -> (18.3388, 54.4068) centre (18.3388, 54.4322) ccw
  arc A1790 (6.6516, 46.5248) -> (6.6998, 46.5408) centre (6.6757, 46.5328) ccw
  arc A1791 (19.4818, 54.4322) -> (19.5326, 54.4322) centre (19.5072, 54.4322) ccw
  arc A1792 (19.1826, 55.0559) -> (19.1826, 55.1067) centre (19.1826, 55.0813) ccw
  arc A1793 (14.4526, 52.2534) -> (14.4018, 52.2534) centre (14.4272, 52.2534) ccw
  arc A1794 (13.5184, 51.9684) -> (13.5184, 52.0192) centre (13.5184, 51.9938) ccw
  line L553 (13.2588, 52.2534) -> (13.2588, 52.5131)
  arc A1795 (13.2588, 52.2534) -> (13.5184, 51.9938) centre (13.5184, 52.2534) ccw
  arc A1796 (13.2842, 52.2534) -> (13.2334, 52.2534) centre (13.2588, 52.2534) ccw
  line L554 (13.9079, 53.3885) -> (13.2588, 53.7779)
  line L555 (14.4272, 52.5131) -> (14.4272, 52.2534)
  arc A1797 (13.2719, 53.7997) -> (13.2457, 53.7562) centre (13.2588, 53.7779) ccw
  arc A1798 (13.8948, 53.3667) -> (13.921, 53.4103) centre (13.9079, 53.3885) ccw
  line L556 (14.4272, 54.3593) -> (13.2588, 54.3593)
  line L557 (13.2588, 54.3593) -> (14.4272, 55.0084)
  arc A1799 (16.9926, 53.5987) -> (16.9418, 53.5987) centre (16.9672, 53.5987) ccw
  arc A1800 (16.7076, 51.9938) -> (16.9672, 52.2534) centre (16.7076, 52.2534) ccw
  line L558 (16.9672, 52.9496) -> (16.9672, 53.5987)
  arc A1801 (11.9126, 52.2534) -> (11.8618, 52.2534) centre (11.8872, 52.2534) ccw
  arc A1802 (15.8242, 52.2534) -> (15.7734, 52.2534) centre (15.7988, 52.2534) ccw
  arc A1803 (14.1676, 52.0192) -> (14.1676, 51.9684) centre (14.1676, 51.9938) ccw
  line L559 (11.8872, 52.9496) -> (11.8872, 53.5987)
  arc A1804 (10.6934, 52.2534) -> (10.7442, 52.2534) centre (10.7188, 52.2534) ccw
  arc A1805 (63.6552, 12.3105) -> (63.6044, 12.3105) centre (63.6298, 12.3105) ccw
  arc A1806 (16.9672, 53.2488) -> (16.9672, 53.2996) centre (16.9672, 53.2742) ccw
  arc A1807 (11.8707, 52.9303) -> (11.9037, 52.969) centre (11.8872, 52.9497) ccw
  line L560 (15.7988, 52.2534) -> (15.7988, 52.5131)
  line L561 (16.9672, 52.5131) -> (16.9672, 52.2534)
  line L562 (16.0584, 52.9496) -> (15.7988, 53.2742)
  arc A1808 (10.7188, 52.2534) -> (10.9784, 51.9938) centre (10.9784, 52.2534) ccw
  arc A1809 (10.9706, 52.9255) -> (10.9863, 52.9738) centre (10.9784, 52.9497) ccw
  line L563 (11.2381, 53.5014) -> (11.8872, 52.9496)
  arc A1810 (14.4272, 52.9736) -> (14.4272, 53.0244) centre (14.4272, 52.999) ccw
  line L564 (14.4272, 55.0084) -> (13.2588, 55.0084)
  arc A1811 (13.2588, 54.3847) -> (13.2588, 54.3339) centre (13.2588, 54.3593) ccw
  arc A1812 (16.9418, 52.9496) -> (16.9926, 52.9496) centre (16.9672, 52.9496) ccw
  arc A1813 (10.7442, 52.5131) -> (10.6934, 52.5131) centre (10.7188, 52.5131) ccw
  arc A1814 (16.9926, 52.2534) -> (16.9418, 52.2534) centre (16.9672, 52.2534) ccw
  arc A1815 (11.0109, 53.5733) -> (11.0109, 53.6241) centre (11.0109, 53.5987) ccw
  line L565 (15.7988, 53.2742) -> (16.9672, 53.2742)
  arc A1816 (13.2465, 54.3815) -> (13.2711, 54.3371) centre (13.2588, 54.3593) ccw
  arc A1817 (14.4395, 54.9862) -> (14.4149, 55.0306) centre (14.4272, 55.0084) ccw
  arc A1818 (10.7442, 53.3066) -> (10.6934, 53.3066) centre (10.7188, 53.3066) ccw
  arc A1819 (63.6044, 10.2362) -> (63.6552, 10.2362) centre (63.6298, 10.2362) ccw
  arc A1820 (63.6552, 9.7197) -> (63.6044, 9.7197) centre (63.6298, 9.7197) ccw
  arc A1821 (11.9126, 53.5987) -> (11.8618, 53.5987) centre (11.8872, 53.5987) ccw
  arc A1822 (11.6276, 51.9684) -> (11.6276, 52.0192) centre (11.6276, 51.9938) ccw
  arc A1823 (10.9784, 52.0192) -> (10.9784, 51.9684) centre (10.9784, 51.9938) ccw
  arc A1824 (11.2545, 53.5207) -> (11.2216, 53.482) centre (11.2381, 53.5014) ccw
  arc A1825 (16.0584, 52.0192) -> (16.0584, 51.9684) centre (16.0584, 51.9938) ccw
  arc A1826 (63.6552, 11.0151) -> (63.6044, 11.0151) centre (63.6298, 11.0151) ccw
  arc A1827 (16.7076, 52.0192) -> (16.7076, 51.9684) centre (16.7076, 51.9938) ccw
  arc A1828 (10.6934, 53.3066) -> (10.7442, 53.3066) centre (10.7188, 53.3066) ccw
  arc A1829 (15.7988, 52.2534) -> (16.0584, 51.9938) centre (16.0584, 52.2534) ccw
  arc A1830 (16.0386, 52.9338) -> (16.0783, 52.9655) centre (16.0585, 52.9497) ccw
  arc A1831 (16.9418, 52.2534) -> (16.9926, 52.2534) centre (16.9672, 52.2534) ccw
  line L566 (16.7076, 51.9938) -> (16.0584, 51.9938)
  line L567 (63.6298, 10.2362) -> (63.6298, 11.0151)
  arc A1832 (11.0109, 53.6241) -> (11.0109, 53.5733) centre (11.0109, 53.5987) ccw
  line L568 (19.5072, 54.4322) -> (18.3388, 54.4322)
  arc A1833 (15.8242, 52.5131) -> (15.7734, 52.5131) centre (15.7988, 52.5131) ccw
  arc A1834 (11.2197, 53.4838) -> (11.2565, 53.5189) centre (11.2381, 53.5014) ccw
  arc A1835 (15.7988, 53.2996) -> (15.7988, 53.2488) centre (15.7988, 53.2742) ccw
  arc A1836 (10.7188, 53.3066) -> (10.9784, 52.9496) centre (11.094, 53.3066) ccw
  arc A1837 (16.0584, 51.9684) -> (16.0584, 52.0192) centre (16.0584, 51.9938) ccw
  arc A1838 (16.7076, 51.9684) -> (16.7076, 52.0192) centre (16.7076, 51.9938) ccw
  line L569 (63.6298, 8.9408) -> (63.6298, 9.7197)
  arc A1839 (10.7442, 52.2534) -> (10.6934, 52.2534) centre (10.7188, 52.2534) ccw
  line L570 (11.6276, 51.9938) -> (10.9784, 51.9938)
  arc A1840 (15.7734, 52.2534) -> (15.8242, 52.2534) centre (15.7988, 52.2534) ccw
  arc A1841 (11.6276, 51.9938) -> (11.8872, 52.2534) centre (11.6276, 52.2534) ccw
  line L571 (63.6298, 11.5316) -> (63.6298, 12.3105)
  arc A1842 (11.0109, 53.5987) -> (10.7188, 53.3066) centre (11.0109, 53.3066) ccw
  arc A1843 (11.8618, 52.9496) -> (11.9126, 52.9496) centre (11.8872, 52.9496) ccw
  arc A1844 (63.6044, 11.5316) -> (63.6552, 11.5316) centre (63.6298, 11.5316) ccw
  arc A1845 (63.6044, 8.9408) -> (63.6552, 8.9408) centre (63.6298, 8.9408) ccw
  line L572 (63.6298, 12.827) -> (63.6298, 13.6059)
  line L573 (68.7098, 8.9408) -> (68.7098, 9.7197)
  arc A1846 (15.8186, 53.29) -> (15.779, 53.2583) centre (15.7988, 53.2742) ccw
  arc A1847 (45.9813, 26.1699) -> (46.0259, 26.1456) centre (46.0036, 26.1577) ccw
  line L574 (45.5168, 27.1408) -> (45.5168, 27.66)
  line L575 (68.7098, 12.827) -> (68.7098, 13.6059)
  arc A1848 (10.9784, 51.9684) -> (10.9784, 52.0192) centre (10.9784, 51.9938) ccw
  line L576 (66.1698, 12.827) -> (66.1698, 13.6059)
  arc A1849 (11.2381, 53.5014) -> (11.0109, 53.5987) centre (11.011, 53.285) ccw
  arc A1850 (45.5422, 26.2876) -> (45.4914, 26.2876) centre (45.5168, 26.2876) ccw
  arc A1851 (45.5168, 27.1662) -> (45.5168, 27.1154) centre (45.5168, 27.1408) ccw
  arc A1852 (46.6852, 27.1154) -> (46.6852, 27.1662) centre (46.6852, 27.1408) ccw
  arc A1853 (46.5229, 25.9955) -> (46.6852, 26.385) centre (46.1367, 26.385) ccw
  arc A1854 (46.505, 26.0135) -> (46.5408, 25.9775) centre (46.5229, 25.9955) ccw
  arc A1855 (46.6598, 26.385) -> (46.7106, 26.385) centre (46.6852, 26.385) ccw
  arc A1856 (46.1765, 26.5277) -> (46.2203, 26.5019) centre (46.1984, 26.5148) ccw
  line L577 (10.7188, 52.2534) -> (10.7188, 52.5131)
  arc A1857 (66.1952, 12.3105) -> (66.1444, 12.3105) centre (66.1698, 12.3105) ccw
  arc A1858 (66.1952, 9.7197) -> (66.1444, 9.7197) centre (66.1698, 9.7197) ccw
  arc A1859 (66.1952, 13.6059) -> (66.1444, 13.6059) centre (66.1698, 13.6059) ccw
  arc A1860 (46.4256, 26.6192) -> (46.4256, 26.67) centre (46.4256, 26.6446) ccw
  line L578 (68.7098, 11.5316) -> (68.7098, 12.3105)
  arc A1861 (68.6844, 11.5316) -> (68.7352, 11.5316) centre (68.7098, 11.5316) ccw
  arc A1862 (45.7764, 26.028) -> (46.0036, 26.1578) centre (45.7764, 26.2917) ccw
  arc A1863 (45.6345, 26.5645) -> (45.5938, 26.5949) centre (45.6142, 26.5797) ccw
  arc A1864 (68.6844, 10.2362) -> (68.7352, 10.2362) centre (68.7098, 10.2362) ccw
  line L579 (63.6298, 14.1224) -> (63.6298, 14.9013)
  line L580 (68.7098, 10.2362) -> (68.7098, 11.0151)
  arc A1865 (66.1952, 11.0151) -> (66.1444, 11.0151) centre (66.1698, 11.0151) ccw
  arc A1866 (68.7352, 13.6059) -> (68.6844, 13.6059) centre (68.7098, 13.6059) ccw
  arc A1867 (66.1444, 14.1224) -> (66.1952, 14.1224) centre (66.1698, 14.1224) ccw
  arc A1868 (68.6844, 12.827) -> (68.7352, 12.827) centre (68.7098, 12.827) ccw
  arc A1869 (68.7352, 9.7197) -> (68.6844, 9.7197) centre (68.7098, 9.7197) ccw
  arc A1870 (63.6044, 14.1224) -> (63.6552, 14.1224) centre (63.6298, 14.1224) ccw
  line L581 (66.1698, 10.2362) -> (66.1698, 11.0151)
  arc A1871 (45.5422, 27.66) -> (45.4914, 27.66) centre (45.5168, 27.66) ccw
  line L582 (46.1984, 26.5148) -> (46.0036, 26.1578)
  arc A1872 (66.1444, 11.5316) -> (66.1952, 11.5316) centre (66.1698, 11.5316) ccw
  arc A1873 (46.7106, 26.385) -> (46.6598, 26.385) centre (46.6852, 26.385) ccw
  line L583 (66.1698, 11.5316) -> (66.1698, 12.3105)
  arc A1874 (46.6852, 26.385) -> (46.4256, 26.6446) centre (46.4256, 26.385) ccw
  arc A1875 (68.7352, 11.0151) -> (68.6844, 11.0151) centre (68.7098, 11.0151) ccw
  arc A1876 (68.7352, 12.3105) -> (68.6844, 12.3105) centre (68.7098, 12.3105) ccw
  line L584 (66.1698, 8.9408) -> (66.1698, 9.7197)
  arc A1877 (68.7352, 14.9013) -> (68.6844, 14.9013) centre (68.7098, 14.9013) ccw
  arc A1878 (45.6142, 26.5797) -> (45.5168, 26.2876) centre (46.0036, 26.2876) ccw
  arc A1879 (66.1952, 14.9013) -> (66.1444, 14.9013) centre (66.1698, 14.9013) ccw
  arc A1880 (45.7764, 26.0533) -> (45.7764, 26.0026) centre (45.7764, 26.028) ccw
  arc A1881 (63.6552, 13.6059) -> (63.6044, 13.6059) centre (63.6298, 13.6059) ccw
  arc A1882 (16.9926, 52.5131) -> (16.9418, 52.5131) centre (16.9672, 52.5131) ccw
  arc A1883 (11.9126, 52.5131) -> (11.8618, 52.5131) centre (11.8872, 52.5131) ccw
  arc A1884 (63.6552, 14.9013) -> (63.6044, 14.9013) centre (63.6298, 14.9013) ccw
  line L585 (46.6852, 27.1408) -> (45.5168, 27.1408)
  line L586 (68.7098, 14.1224) -> (68.7098, 14.9013)
  arc A1885 (46.7106, 27.66) -> (46.6598, 27.66) centre (46.6852, 27.66) ccw
  arc A1886 (45.4914, 26.2876) -> (45.5422, 26.2876) centre (45.5168, 26.2876) ccw
  arc A1887 (66.1444, 10.2362) -> (66.1952, 10.2362) centre (66.1698, 10.2362) ccw
  arc A1888 (11.6276, 52.0192) -> (11.6276, 51.9684) centre (11.6276, 51.9938) ccw
  arc A1889 (46.4256, 26.67) -> (46.4256, 26.6192) centre (46.4256, 26.6446) ccw
  arc A1890 (45.4914, 27.1408) -> (45.5422, 27.1408) centre (45.5168, 27.1408) ccw
  arc A1891 (63.6044, 12.827) -> (63.6552, 12.827) centre (63.6298, 12.827) ccw
  line L587 (46.0361, 27.1408) -> (46.0361, 27.5302)
  line L588 (66.1698, 14.1224) -> (66.1698, 14.9013)
  arc A1892 (66.1444, 12.827) -> (66.1952, 12.827) centre (66.1698, 12.827) ccw
  arc A1893 (46.2207, 26.5026) -> (46.1761, 26.5269) centre (46.1984, 26.5148) ccw
  line L589 (46.6852, 27.66) -> (46.6852, 27.1408)
  line L590 (48.5902, 28.091) -> (47.4218, 28.091)
  arc A1894 (45.8414, 30.4405) -> (45.8414, 30.3897) centre (45.8414, 30.4151) ccw
  arc A1895 (47.4416, 29.6125) -> (47.402, 29.5808) centre (47.4218, 29.5966) ccw
  arc A1896 (46.0107, 27.1408) -> (46.0615, 27.1408) centre (46.0361, 27.1408) ccw
  arc A1897 (45.4914, 28.461) -> (45.5422, 28.461) centre (45.5168, 28.461) ccw
  arc A1898 (45.8414, 31.0896) -> (45.8414, 31.0388) centre (45.8414, 31.0642) ccw
  arc A1899 (47.4472, 28.4155) -> (47.3964, 28.4155) centre (47.4218, 28.4155) ccw
  arc A1900 (46.3606, 30.3897) -> (46.3606, 30.4405) centre (46.3606, 30.4151) ccw
  line L591 (47.7464, 28.7401) -> (48.2656, 28.7401)
  arc A1901 (47.4218, 29.622) -> (47.4218, 29.5712) centre (47.4218, 29.5966) ccw
  line L592 (48.5902, 29.2721) -> (48.5902, 29.9212)
  arc A1902 (45.5168, 28.1619) -> (45.5168, 28.1111) centre (45.5168, 28.1365) ccw
  arc A1903 (66.1444, 8.9408) -> (66.1952, 8.9408) centre (66.1698, 8.9408) ccw
  arc A1904 (45.5168, 26.2876) -> (45.7764, 26.028) centre (45.7764, 26.2876) ccw
  arc A1905 (46.3606, 30.4405) -> (46.3606, 30.3897) centre (46.3606, 30.4151) ccw
  line L593 (46.6852, 29.5966) -> (45.5168, 29.9861)
  arc A1906 (47.3964, 28.4155) -> (47.4472, 28.4155) centre (47.4218, 28.4155) ccw
  line L594 (48.5902, 28.4155) -> (48.5902, 28.091)
  arc A1907 (45.4914, 28.1365) -> (45.5422, 28.1365) centre (45.5168, 28.1365) ccw
  arc A1908 (46.0255, 26.1449) -> (45.9818, 26.1707) centre (46.0037, 26.1578) ccw
  arc A1909 (48.5648, 28.4156) -> (48.6156, 28.4155) centre (48.5902, 28.4155) ccw
  line L595 (46.6852, 28.1365) -> (45.5168, 28.1365)
  arc A1910 (47.7464, 28.7147) -> (47.7464, 28.7655) centre (47.7464, 28.7401) ccw
  line L596 (45.5168, 29.2072) -> (46.6852, 29.5966)
  arc A1911 (45.5248, 30.0102) -> (45.5088, 29.962) centre (45.5168, 29.9861) ccw
  arc A1912 (46.4256, 26.6446) -> (46.1984, 26.5148) centre (46.4256, 26.3809) ccw
  arc A1913 (47.7464, 28.7401) -> (47.4218, 28.4155) centre (47.7464, 28.4155) ccw
  arc A1914 (48.5902, 28.0656) -> (48.5902, 28.1164) centre (48.5902, 28.091) ccw
  arc A1915 (46.6932, 29.5726) -> (46.6772, 29.6207) centre (46.6852, 29.5967) ccw
  arc A1916 (46.1405, 28.1365) -> (46.1913, 28.1365) centre (46.1659, 28.1365) ccw
  arc A1917 (46.6598, 27.1408) -> (46.7106, 27.1408) centre (46.6852, 27.1408) ccw
  arc A1918 (46.6852, 28.1111) -> (46.6852, 28.1619) centre (46.6852, 28.1365) ccw
  line L597 (47.4218, 28.091) -> (47.4218, 28.4155)